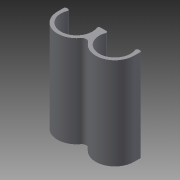
# Autodesk Inventor part: spool holder
Saved by Autodesk Inventor 2013 (Build 170138000, 138)
## iProperties
Created: 2012-12-18
Part Number: spool holder
Material: Generic
Document SubType Name: Modeling
Designer: Tars
Density: 1 g/cm^3
Author: Tars
Autodesk Inventor part; units mm, degrees
ref_plane "YZ Plane" through (0, 0, 0) normal (1, 0, 0) x (0, 1, 0)
ref_plane "XZ Plane" through (0, 0, 0) normal (0, 1, 0) x (-1, 0, 0)
ref_plane "XY Plane" through (0, 0, 0) normal (0, 0, 1) x (1, 0, 0)
sketch "Sketch1" plane through (0, 0, 0) normal (0, 0, 1) x (1, 0, 0)
  arc A0 (-25, 0) -> (0, 0) centre (-12.5, 0) ccw construction
  arc A1 (0, 0) -> (25, 0) centre (12.5, 0) ccw construction
  line L0 (-25, 0) -> (25, 0) construction
  line L1 (-25, 0) -> (-25, 4)
  line L2 (25, 0) -> (25, 4)
  arc A2 (-22.0802, 3.6444) -> (-2.9198, 3.6444) centre (-12.5, 0) ccw
  arc A3 (2.9198, 3.6444) -> (22.0802, 3.6444) centre (12.5, 0) ccw
  line L3 (-24, 5) -> (-23.0149, 5)
  line L4 (-1.9851, 5) -> (1.9851, 5)
  line L5 (23.0149, 5) -> (24, 5)
  arc A4 (2.4194, -7.3913) -> (-2.4194, -7.3913) centre (0, -9.1652) ccw
  arc A5 (-22.0802, 3.6444) -> (-23.0149, 5) centre (-23.0149, 4) ccw
  arc A6 (-24, 5) -> (-25, 4) centre (-24, 4) ccw
  arc A7 (-1.9851, 5) -> (-2.9198, 3.6444) centre (-1.9851, 4) ccw
  arc A8 (2.9198, 3.6444) -> (1.9851, 5) centre (1.9851, 4) ccw
  arc A9 (23.0149, 5) -> (22.0802, 3.6444) centre (23.0149, 4) ccw
  arc A10 (25, 4) -> (24, 5) centre (24, 4) ccw
  arc A11 (-25, 0) -> (-2.4194, -7.3913) centre (-12.5, 0) ccw
  arc A12 (2.4194, -7.3913) -> (25, 0) centre (12.5, 0) ccw
  line L6 (-24, 5) -> (-23.0149, 5)
  point P0 (25, 5)
  point P1 (-3.5522, 5)
  point P2 (3.5522, 5)
  point P3 (21.4478, 5)
  dimension "d0" = 12.5
  dimension "d2" = 12.5
  dimension "d3" = 5
  dimension "d5" = 10.25
  dimension "d6" = 10.25
  dimension "d9" = 3
  dimension "d10" = 1
  dimension "d11" = 1
  constraints: 31 point on circle, 22 tangent, 14 end point, 13 centre point, 11 point on line, 4 equal radius, 3 collinear, 2 concentric, 2 horizontal, 1 midpoint, 1 parallel, 1 perpendicular
  measures "d0" radius of A0
  measures "d2" radius of A1
  measures "d3" distance of L0.end point (25, 5)
  measures "d5" radius of A2
  measures "d6" radius of A3
  measures "d9" radius of A4
  measures "d10" radius of A5
  measures "d11" radius of A6
extrude "Extrusion2" add sketch "Sketch1" along normal blind 60
equation "\"d2\" = d0"
equation "\"d6\" = d5"
body "Solid2"
